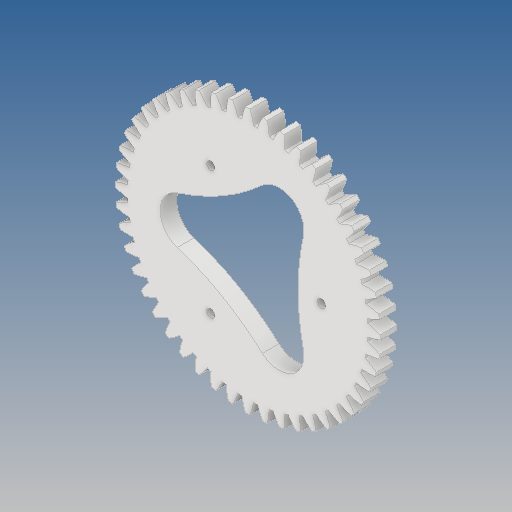
# Autodesk Inventor part: engrane acrílico C
Saved by Autodesk Inventor 2017 (Build 210142000, 142)
## iProperties
Part Number: engrane acrílico C
Material: Genérico
Document SubType Name: Modeling
Designer: FABLAB
Density: 1 g/cm^3
Appearance: Blanco
Author: FABLAB
Autodesk Inventor part; units mm, degrees
ref_plane "YZ Plane" through (0, 0, 0) normal (1, 0, 0) x (0, 1, 0)
ref_plane "XZ Plane" through (0, 0, 0) normal (0, 1, 0) x (-1, 0, 0)
ref_plane "XY Plane" through (0, 0, 0) normal (0, 0, 1) x (1, 0, 0)
sketch "Boceto1" plane through (0, 0, 0) normal (0, 0, 1) x (1, 0, 0)
  circle A0 centre (-13.375, 23.1662) radius 1.5 projected
  circle A1 centre (-13.375, -23.1662) radius 1.5 projected
  circle A2 centre (26.75, 0) radius 1.5 projected
  arc A3 (20.168, 17.783) -> (20.168, -17.783) centre (101.6471, 0) ccw projected
  arc A4 (5.3165, -26.3575) -> (20.168, -17.783) centre (11.375, -19.7021) ccw projected
  arc A5 (5.3165, -26.3575) -> (-25.4845, -8.5745) centre (-50.8235, -88.0289) ccw projected
  arc A6 (-25.4845, 8.5745) -> (-25.4845, -8.5745) centre (-22.75, 0) ccw projected
  arc A7 (-25.4845, 8.5745) -> (5.3165, 26.3575) centre (-50.8235, 88.0289) ccw projected
  arc A8 (20.168, 17.783) -> (5.3165, 26.3575) centre (11.375, 19.7021) ccw projected
  circle A9 centre (0, 0) radius 45 construction
  circle A10 centre (0, 0) radius 57
  point P0 (0, 0)
  dimension "d0" = 114
  constraints: 1 centre point, 1 coincident
  measures "d0" diameter of A10
extrude "Extrusión1" add sketch "Boceto1" along normal blind 6
spur gear teeth "Engranaje recto2" teeth 48 pitch diameter 96 tip diameter 96 root diameter 87 face width 7 trims to tip circle yes start plane through (0, 0, 0) normal (0, 0, -1) x (-1, 0, 0)
